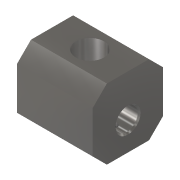
# Autodesk Inventor part: 10-004-ACTR-FIX
Saved by Autodesk Inventor 2018 (Build 220112000, 112)
## iProperties
Created: 2017-07-23
Part Number: 10-004-ACTR-FIX
Material: Stainless Steel
Document SubType Name: Modeling
Designer: Martin Fees
Density: 8 g/cm^3
Appearance: Semi-Polished
Author: Martin Fees
Autodesk Inventor part; units mm, degrees
note: some values were not read from the file. Chosen so that the rebuilt part matches the saved one: direction of "Hole_Wheel_Fix".
ref_plane "YZ Plane" through (0, 0, 0) normal (1, 0, 0) x (0, 1, 0)
ref_plane "XZ Plane" through (0, 0, 0) normal (0, 1, 0) x (-1, 0, 0)
ref_plane "XY Plane" through (0, 0, 0) normal (0, 0, 1) x (1, 0, 0)
sketch "Sketch1" plane through (0, 0, 0) normal (1, 0, 0) x (0, 1, 0)
  line L0 (0, 35) -> (0, -35) projected
  line L1 (-35, 0) -> (35, 0) projected
  line L2 (-25, -25) -> (25, -25)
  line L3 (25, -25) -> (25, 25)
  line L4 (25, 25) -> (-25, 25)
  line L5 (-25, 25) -> (-25, -25)
  line L6 (-25, -25) -> (25, 25) construction
  line L7 (25, -25) -> (-25, 25) construction
  point P0 (0, 0)
  dimension "d1" = 50
  dimension "d2" = 50
  constraints: 12 end point, 2 midpoint, 2 parallel, 1 horizontal, 1 perpendicular
  measures "d1" distance of L2.end L3.end
  measures "d2" distance of L3.end L4.end
extrude "Base" add sketch "Sketch1" along normal mid plane 54
sketch "Sketch2" plane through (27, 0, 0) normal (1, 0, 0) x (0, 0, -1)
  line L0 (-35, 0) -> (35, 0) construction
  line L1 (25, -25) -> (25, 25) construction
  point P0 (0, 0)
  point P1 (5, 0)
  dimension "d5" = 20
  constraints: 1 point on line
  measures "d5" distance from line of L1 point (5, 0)
hole "Hole_Wheel" at (27, 0, -5) direction (-1, 0, 0) diameter 16 end through all
sketch "Sketch3" plane through (27, 25, -25) normal (0, 0, -1) x (-1, 0, 0)
  line L0 (54, -33) -> (0, -33) construction
  line L1 (54, -17) -> (0, -17) construction
  line L2 (54, 0) -> (0, 0) construction
  line L3 (0, -50) -> (0, 0) construction
  line L4 (0, -50) -> (54, -50) construction
  line L5 (54, 0) -> (54, -50) construction
  line L6 (54, -50) -> (54, 0) projected
  line L7 (54, -25) -> (0, -25) construction
  line L8 (54, -50) -> (0, -50) projected
  line L9 (27, -50) -> (27, 0) construction
  line L10 (54, 0) -> (0, 0) projected
  point P0 (27, -25)
  point P1 (44.5, -25)
  point P2 (9.5, -25)
  point P3 (27, -25)
  dimension "d13" = 35
  constraints: 4 end point, 4 midpoint, 2 point on line, 1 coincident, 1 symmetric about line
  measures "d13" distance of point (9.5, -25) point (44.5, -25)
hole "Hole_Wheel_Fix" at (-17.5, 0, -25) at (17.5, 0, -25) at (0, 0, -25) direction (0, 0, 1) diameter 4.459 end up to surface countersink diameter 11.5 countersink angle 90 thread size "M5x0.5" class "6H" standard "ISO Metric profile"
sketch "Sketch4" plane through (-27, -25, 25) normal (0, 0, 1) x (1, 0, 0)
  line L0 (54, 50) -> (54, 0) construction
  line L1 (0, 0) -> (0, 50) construction
  line L2 (0, 50) -> (54, 50) construction
  line L3 (0, 0) -> (54, 0) construction
  line L4 (54, 0) -> (54, 50) construction
  line L5 (52, 52) -> (0, 0) construction
  line L6 (54, 0) -> (0, 0) construction
  line L7 (52, -2) -> (0, 50) construction
  point P0 (27, 25)
  point P1 (27, 25)
  constraints: 4 end point, 1 coincident, 1 perpendicular
hole "ConnectionPipe" at (0, 0, 25) direction (0, 0, -1) diameter 20 depth 15 tip angle 118
chamfer "Chamfer1" distance 10 angle 45 4 edges at (0, 25, -25) (0, -25, -25) (0, 25, 25) (0, -25, 25)
chamfer "Chamfer2" distance 1 angle 45 2 edges at (-27, 0, 3) (27, 0, 3)
body "Solid1"
